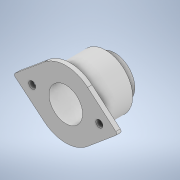
# Autodesk Inventor part: Bearing Block WCP
Saved by Autodesk Inventor 2020 (Build 240168000, 168)
## iProperties
Created: 2020-01-16
Part Number: Bearing Block WCP
Material: Generic
Document SubType Name: Modeling
Designer: aidan
Density: 1 g/cm^3
Appearance: Default
Author: aidan
Autodesk Inventor part; units mm, degrees
ref_plane "YZ Plane" through (0, 0, 0) normal (1, 0, 0) x (0, 1, 0)
ref_plane "XZ Plane" through (0, 0, 0) normal (0, 1, 0) x (-1, 0, 0)
ref_plane "XY Plane" through (0, 0, 0) normal (0, 0, 1) x (1, 0, 0)
sketch "Sketch2" plane through (0, 0, 0) normal (0, 0, 1) x (1, 0, 0)
  arc A0 (-35.8105, 1.2215) -> (-35.8105, -1.2215) centre (-34.7965, 0) ccw
  arc A1 (35.4376, -1.3856) -> (35.4495, 1.0387) centre (34.4185, -0.1685) ccw
  line L0 (-35.8105, 1.2215) -> (-15.2094, 18.3224)
  line L1 (-35.8105, -1.2215) -> (-15.2094, -18.3224)
  line L2 (-73.8497, 0) -> (129.1726, 0) construction
  line L3 (15.465, 18.1071) -> (35.4495, 1.0387)
  line L4 (35.4376, -1.3856) -> (15.2871, -18.2576)
  line L5 (-36.384, 17.9881) -> (-36.384, -16.5847) construction
  line L6 (36.006, 40.1283) -> (36.006, -35.2466) construction
  circle A2 centre (-23.8125, 0) radius 2.4892
  circle A3 centre (23.8125, 0) radius 2.4892
  circle A4 centre (0, 0) radius 11.8999
  arc A5 (-15.2094, -18.3224) -> (15.2871, -18.2576) centre (0, 0) ccw
  arc A6 (15.465, 18.1071) -> (-15.2094, 18.3224) centre (0, 0) ccw
  dimension "d6" = 3.175
  dimension "d7" = 72.39
  dimension "d8" = 23.7998
  dimension "d9" = 4.9784
  constraints: 14 end point, 10 tangent, 8 point on circle, 7 centre point, 4 point on line, 2 coincident, 2 equal radius, 2 vertical, 1 horizontal
  measures "d6" diameter of A0
  measures "d7" distance between parallel lines of L5 L6
  measures "d8" diameter of A4
  measures "d9" diameter of A2
extrude "Extrusion1" add sketch "Sketch2" along normal blind 3.175
sketch "Sketch3" plane through (0, 0, 0) normal (0, 0, -1) x (-1, 0, 0)
  circle A0 centre (0, 0) radius 19.05
  circle A1 centre (0, 0) radius 11.8999 projected
  dimension "d12" = 38.1
  constraints: 1 centre point, 1 coincident
  measures "d12" diameter of A0
extrude "Extrusion2" add sketch "Sketch3" along normal blind 25.146
sketch "Sketch4" plane through (0, 0, -25.146) normal (0, 0, -1) x (-1, 0, 0)
  circle A0 centre (0, 0) radius 11.8999 projected
  circle A1 centre (0, 0) radius 14.2621
  dimension "d15" = 28.5242
  constraints: 1 centre point, 1 coincident
  measures "d15" diameter of A1
extrude "Extrusion3" add sketch "Sketch4" along normal blind 6.35
body "Solid1"
